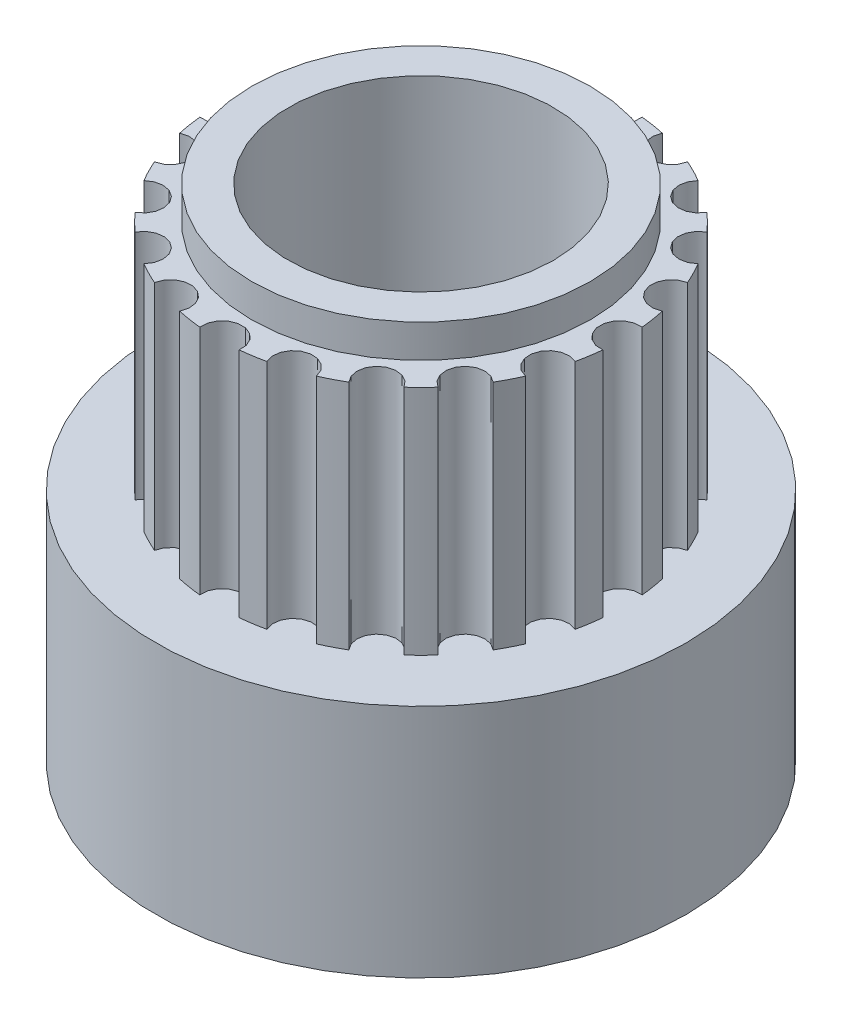
# Autodesk Inventor part: GT2Pulley_20T_8mm
Saved by Autodesk Inventor 2022 (Build 260153000, 153)
## iProperties
Created: 2021-10-20
Part Number: GT2Pulley_20T_8mm
Material: Generic
Document SubType Name: Modeling
Designer: DDeGo
Density: 1 g/cm^3
Appearance: Default
Author: DDeGo
Autodesk Inventor part; units mm, degrees
ref_plane "YZ Plane" through (0, 0, 0) normal (1, 0, 0) x (0, 1, 0)
ref_plane "XZ Plane" through (0, 0, 0) normal (0, 1, 0) x (-1, 0, 0)
ref_plane "XY Plane" through (0, 0, 0) normal (0, 0, 1) x (1, 0, 0)
sketch "Sketch1" plane through (0, 0, 0) normal (0, 0, 1) x (1, 0, 0)
  line L0 (0, 0) -> (4, 0) construction
  line L1 (8, 0) -> (8, 7.1)
  line L2 (8, 7.1) -> (6.11, 7.1)
  line L3 (6.11, 7.1) -> (6.11, 14.1)
  line L4 (6.11, 14.1) -> (5.11, 14.1)
  line L5 (5.11, 14.1) -> (5.11, 15.1)
  line L6 (5.11, 15.1) -> (4, 15.1)
  line L7 (0, 15.1) -> (0, 0) construction
  line L8 (4, 15.1) -> (4, 0)
  line L9 (4, 15.1) -> (0, 15.1) construction
  line L10 (4, 0) -> (8, 0)
  dimension "d0" = 7
  dimension "d1" = 7.1
  dimension "d2" = 8
  dimension "d3" = 6.11
  dimension "d5" = 1
  dimension "d6" = 1
  dimension "d15" = 4
  constraints: 22 end point, 10 perpendicular, 2 horizontal, 1 vertical
  measures "d0" distance of L2.end L3.end
  measures "d1" distance of L1.start L1.end
  measures "d2" distance between parallel lines of L1 L7
  measures "d3" distance between parallel lines of L7 L3
  measures "d5" distance of L4.end L5.end
  measures "d6" distance of L3.end L4.end
  measures "d15" distance between parallel lines of L7 L8
revolve "Revolution1" add sketch "Sketch1" angle 360 about axis through (0, 15.1, 0) along (0, -1, 0)
sketch "Sketch2" plane through (0, 14.1, 0) normal (0, 1, 0) x (1, 0, 0)
  circle A0 centre (0, 0) radius 5.11 construction
  line L0 (0, 0) -> (-6, 0) construction
  circle A1 centre (-6, 0) radius 0.6
  point P0 (0, 0)
  dimension "d8" = 1.2
  dimension "d9" = 6
  constraints: 2 end point, 1 centre point, 1 coincident, 1 horizontal
  measures "d8" diameter of A1
  measures "d9" distance of L0.start L0.end
extrude "Extrusion1" cut sketch "Sketch2" against normal up to surface (7 mm away)
pattern_circular "Circular Pattern1" count 20 over 360 about axis through (0, 14.6, 0) along (0, -1, 0) of "Extrusion1"
sketch "Sketch3" plane through (0, 0, 0) normal (1, 0, 0) x (0, 1, 0)
  line L0 (7.1, 8) -> (7.1, -8) construction
  line L1 (0, 8) -> (0, -8) construction
  line L2 (0, 0) -> (7.1, 0) construction
  circle A0 centre (3.55, 0) radius 1.25
  dimension "d16" = 2.5
  constraints: 2 end point, 2 midpoint, 1 centre point
  measures "d16" diameter of A0
extrude "Extrusion2" cut sketch "Sketch3" against normal blind 10
pattern_circular "Circular Pattern2" count 2 over 90 about axis through (0, 7.55, 0) along (0, -1, 0) of "Extrusion2"
body "Solid1"
